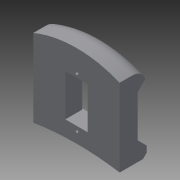
# Autodesk Inventor part: servodrzak
Saved by Autodesk Inventor 2015 (Build 190159000, 159)
## iProperties
Created: 2015-03-15
Part Number: servodrzak
Material: Generic
Document SubType Name: Modeling
Designer: Turboslimak
Density: 1 g/cm^3
Appearance: Default
Author: Turboslimak
Autodesk Inventor part; units mm, degrees
ref_plane "YZ Plane" through (0, 0, 0) normal (1, 0, 0) x (0, 1, 0)
ref_plane "XZ Plane" through (0, 0, 0) normal (0, 1, 0) x (-1, 0, 0)
ref_plane "XY Plane" through (0, 0, 0) normal (0, 0, 1) x (1, 0, 0)
sketch "Sketch1" plane through (0, 0, 0) normal (0, 1, 0) x (-1, 0, 0)
  line L0 (23.95, 58.2495) -> (23.95, 15)
  line L1 (-24.05, 15) -> (-24.05, 58.2495)
  line L2 (23.95, 58.2495) -> (23.95, 15)
  arc A0 (23.95, 58.2495) -> (-24.05, 58.2495) centre (-0.05, 0) ccw
  arc A1 (23.95, 15) -> (-24.05, 15) centre (-0.05, -133.0676) ccw
  line L3 (-0.05, 25.518) -> (-0.05, 48.718)
  line L4 (-6.25, 25.518) -> (6.15, 25.518)
  line L5 (6.15, 25.518) -> (6.15, 48.718)
  line L6 (6.15, 48.718) -> (-6.25, 48.718)
  line L7 (-6.25, 48.718) -> (-6.25, 25.518)
  line L8 (-6.25, 25.518) -> (6.15, 48.718) construction
  line L9 (6.15, 25.518) -> (-6.25, 48.718) construction
  line L10 (23.95, 15) -> (23.95, 58.2495)
  line L11 (-24.05, 15) -> (-24.05, 58.2495)
  arc A2 (23.95, 15) -> (-24.05, 15) centre (-0.05, -133.0676) ccw
  arc A3 (23.95, 58.2495) -> (-24.05, 58.2495) centre (-0.05, 0) ccw
  point P0 (-0.05, 37.118)
  dimension "d6" = 150
  dimension "d7" = 23.2
  dimension "d8" = 12.4
  constraints: 24 end point, 8 point on circle, 5 equal length, 4 centre point, 3 midpoint, 1 concentric, 1 horizontal, 1 perpendicular
  measures "d6" radius of A1
  measures "d7" distance of L3.start L3.end
  measures "d8" distance of L6.end L5.end
extrude "Extrusion1" add sketch "Sketch1" along normal blind 15
sketch "Sketch2" plane through (0, 15, 0) normal (0, 1, 0) x (1, 0, 0)
  line L0 (-6.15, -48.718) -> (6.25, -48.718)
  line L1 (6.25, -48.718) -> (6.25, -25.518)
  line L2 (6.25, -25.518) -> (-6.15, -25.518)
  line L3 (-6.15, -25.518) -> (-6.15, -48.718)
  line L4 (24.05, -58.2495) -> (24.05, -15) projected
  line L5 (-24.0098, -48.718) -> (24.05, -48.718)
  line L6 (24.05, -48.718) -> (24.05, -25.518)
  line L7 (24.05, -25.518) -> (-24.0098, -25.518)
  line L8 (-24.0098, -25.518) -> (-24.0098, -48.718)
  point P0 (0, 0)
  constraints: 16 end point, 4 parallel, 3 point on line, 2 horizontal, 2 perpendicular
extrude "Extrusion2" cut sketch "Sketch2" against normal blind 5 contours L5 L8 L7 L3 | L1 L7 L4 L5
sketch "Sketch3" plane through (0, 0, 0) normal (0, -1, 0) x (1, 0, 0)
  line L0 (24.05, 48.718) -> (-23.95, 48.718) projected
  line L1 (0.05, 48.718) -> (0.05, 51.068)
  circle A0 centre (0.05, 51.068) radius 1
  line L2 (-23.95, 25.518) -> (24.05, 25.518) projected
  line L3 (0.05, 25.518) -> (0.05, 23.168)
  circle A1 centre (0.05, 23.168) radius 1
  point P0 (0, 0)
  dimension "d13" = 2.35
  dimension "d14" = 2
  dimension "d15" = 2.35
  dimension "d16" = 2
  constraints: 4 end point, 2 centre point, 2 coincident, 2 midpoint, 2 vertical
  measures "d13" distance of L1.start L1.end
  measures "d14" diameter of A0
  measures "d15" distance of L3.start L3.end
  measures "d16" diameter of A1
extrude "Extrusion3" cut sketch "Sketch3" against normal blind 5
fillet "Fillet1" radius 8 1 edges at (0.05, 15, 63)
chamfer "Chamfer1" distance 5 angle 45 2 edges at (0.05, 15, 48.718) (0.05, 15, 25.518)
chamfer "Chamfer2" distance 2 angle 45 1 edges at (0.05, 15, 16.9324)
fillet "Fillet2" radius 1 2 edges at (6.25, 10, 37.118) (-6.15, 10, 37.118)
fillet "Fillet3" radius 1 3 edges at (-17.8761, 14.8588, 53.5769) (0.05, 15, 53.718) (17.9761, 14.8588, 53.5769)
body "Solid1"
